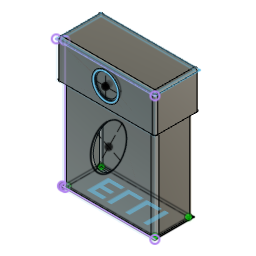
Kartenbox (Autodesk Fusion 360 design; units mm, degrees)
Autodesk Fusion 360 part; units mm, degrees
sketch "Sketch1" plane through (0, 0, 0) normal (0, 0, 1) x (1, 0, 0) in component "Component"
  line L0 (0, 0) -> (69, 0)
  line L1 (69, 0) -> (69, 29)
  line L2 (69, 29) -> (0, 29)
  line L3 (0, 29) -> (0, 0)
  line L4 (2, 27) -> (67, 27)
  line L5 (67, 27) -> (67, 2)
  line L6 (67, 2) -> (2, 2)
  line L7 (2, 2) -> (2, 27)
  line L8 (2, 27) -> (67, 27) construction
  line L9 (67, 27) -> (67, 2) construction
  line L10 (67, 2) -> (2, 2) construction
  line L11 (2, 2) -> (2, 27) construction
  dimension "d46" = 2
  dimension "d47" = 2
  dimension "d48" = 2
  dimension "d49" = 2
  dimension "d80" = 25
  dimension "d81" = 65
  dimension "d98" = 16
  text T0 "ELLI" font "Arial" height 16 bold align centre middle in box 65 x 25 at (2, 27) x (1, 0) y (0, -1) spacing 1 kerned
  constraint horizontal L0
  constraint vertical L1
  constraint horizontal L2
  constraint vertical L3
  constraint coincident L0.start L3.end
  constraint horizontal L4
  constraint vertical L5
  constraint horizontal L6
  constraint vertical L7
  constraint coincident L6.end
  constraint collinear L4 L8
  constraint collinear L5 L9
  measures "d46" distance of L2 L4
  measures "d47" distance of L0 L6
  measures "d48" distance of L3 L7
  measures "d49" distance of L1 L5
  measures "d80" distance of L4 L6
  measures "d81" distance of L5 L7
extrude "Extrude1" add sketch "Sketch1" along normal blind 95 makes body 1 in component "Component"
extrude "Extrude2" add sketch "Sketch1" against normal blind 2 contours L0 L1 L2 L3 | L4 L5 L6 L7 bodies 1 in component "Component"
sketch "Sketch2" plane through (0, 0, 0) normal (0, -1, 0) x (1, 0, 0) in component "Component"
  line L0 (69, -2) -> (69, 95)
  line L1 (69, 95) -> (0, 95)
  line L2 (0, 95) -> (0, -2)
  line L3 (0, -2) -> (69, -2)
  circle A0 centre (34.5, 83) radius 9
  ellipse E0 centre (34.5, 42.5) end of major axis (44.5, 62.6556) minor radius 10
  line L4 (24.5, 22.3444) -> (44.5, 62.6556)
  line L5 (43.4581, 38.0556) -> (25.5419, 46.9444)
  line L6 (2, 0) -> (2, 95)
  line L7 (0, 0) -> (69, 0)
  dimension "d67" = 18
  dimension "d69" = 12
  dimension "d93" = 34.5
  dimension "d94" = 42.5
  dimension "d95" = 45
  dimension "d96" = 20
  dimension "d97" = 10
  constraint coincident E0 L4.start
  constraint coincident E0 L4.end
  constraint coincident E0 L5.start
  constraint coincident E0 L5.end
  constraint vertical A0.centre E0.centre
  measures "d67" diameter of A0
  measures "d69" distance of L1 A0.centre
  measures "d93" distance of L2 A0.centre
  measures "d94" distance of E0.centre L7
  measures "d95" distance of E0
  measures "d97" distance of E0.centre L4.end
extrude "Extrude3" add sketch "Sketch2" along normal blind 1 contours A0 bodies 1 in component "Component"
draft "Draft1" angle 1.5 neutral plane through (0, 0, 95) pull (0, 0, 1) 1 faces at (37.1694, -1, 83.8545) on bodies 1 in component "Component"
extrude "Extrude4" add sketch "Sketch2" along normal blind -29 and the other way blind 30 contours A0 bodies 1 in component "Component"
draft "Draft2" angle 1.5 neutral plane through (0, 0, 95) pull (0, 0, 1) 1 faces at (37.1694, 30, 83.8545) on bodies 1 in component "Component"
extrude "Extrude5" cut sketch "Sketch2" against normal blind 41.885 contours E0 L4 L5 | E0 L4 L5 | E0 L4 L5 | E0 L4 L5 bodies 1 in component "Component"
extrude "Extrude6" cut sketch "Sketch1" against normal blind 5.147 and the other way blind -1.5 text T0 bodies 1 in component "Component"
fillet "Fillet3" radius 3 8 edges at (69, 29, 46.5) (0, 0, 46.5) (0, 29, 46.5) (0, 14.5, -2) (34.5, 29, -2) (34.5, 0, -2) (69, 14.5, -2) (69, 0, 46.5) on bodies 1 in component "Component"
fillet "Fillet1" radius 1.3 20 edges at (26.1091, 29, 79.7455) (26.1091, 0, 86.2545) (34.5, -1.5499, 74) (34.5, 0, 95) (34.5, 29, 95) (69, 14.5, 95) (0, 14.5, 95) (34.5, 30.0786, 92) (2, 27, 47.5) (2, 2, 47.5) (67, 2, 47.5) (67, 27, 47.5) (34.5, 27, 0) (2, 14.5, 0) (34.5, 2, 0) (67, 14.5, 0) (68.1213, 28.1213, 95) (0.8787, 28.1213, 95) (0.8787, 0.8787, 95) (68.1213, 0.8787, 95) on bodies 1 in component "Component"
sketch "Sketch1 (2)" plane through (0, 0, 0) normal (0, 0, 1) x (1, 0, 0) in component "Component'"
  line L0 (1.3, 23.99) -> (70.95, 23.99)
  line L1 (70.95, 23.99) -> (70.95, -5.3725)
  line L2 (70.95, -5.3725) -> (1.3, -5.3725)
  line L3 (1.3, -5.3725) -> (1.3, 23.99)
  line L4 (-0.7, -7.3725) -> (72.95, -7.3725)
  line L5 (72.95, -7.3725) -> (72.95, 25.99)
  line L6 (72.95, 25.99) -> (-0.7, 25.99)
  line L7 (-0.7, 25.99) -> (-0.7, -7.3725)
  dimension "d56" = 2
  dimension "d57" = 2
  dimension "d58" = 2
  dimension "d59" = 2
  dimension "d82" = 29.3625
  dimension "d83" = 69.65
  constraint horizontal L0
  constraint vertical L1
  constraint horizontal L2
  constraint vertical L3
  constraint horizontal L4
  constraint vertical L5
  constraint horizontal L6
  constraint vertical L7
  measures "d56" distance of L1 L5
  measures "d57" distance of L3 L7
  measures "d58" distance of L2 L4
  measures "d59" distance of L0 L6
  measures "d82" distance of L0.end L1.end
  measures "d83" distance of L0.start L0.end
extrude "Extrude1'" add sketch "Sketch1 (2)" against normal blind 27 separate body makes body 2 in component "Component'"
extrude "Extrude2'" add sketch "Sketch1 (2)" along normal blind 2 contours L0 L1 L2 L3 | L4 L5 L6 L7 bodies 2 in component "Component'"
sketch "Sketch2 (2)" plane through (0, -7.3725, 0) normal (0, -1, 0) x (1, 0, 0) in component "Component'"
  line L0 (-0.7, 2) -> (-0.7, -27)
  line L1 (-0.7, -27) -> (72.95, -27)
  line L2 (72.95, -27) -> (72.95, 2)
  line L3 (72.95, 2) -> (-0.7, 2)
  circle A0 centre (36.125, -12.3) radius 9.25
  line L4 (-0.7, 0) -> (72.95, 0)
  ellipse E0 centre (36.125, -12.3) end of major axis (36.125, -2.85) minor radius 9.25
  line L5 (36.125, -21.75) -> (36.125, -2.85)
  line L6 (45.375, -12.3) -> (26.875, -12.3)
  dimension "d64" = 18.5
  dimension "d68" = 12.3
  dimension "d91" = 36.825
  dimension "d104" = 18.9
  constraint concentric A0 E0
  constraint vertical L5
  constraint coincident E0 L5.start
  constraint coincident E0 L5.end
  constraint coincident E0 L6.start
  constraint coincident E0 L6.end
  constraint coincident A0 L6.start
  measures "d64" diameter of A0
  measures "d68" distance of A0.centre L4
  measures "d91" distance of L0 A0.centre
  measures "d104" distance of E0
extrude "Extrude3'" cut sketch "Sketch2 (2)" against normal blind 49.869 contours A0 L5 L6 | A0 E0 L5 | A0 E0 L5 | A0 L5 L6 | A0 L5 L6 | A0 E0 L5 | A0 E0 L5 | A0 L5 L6 bodies 2 in component "Component'"
fillet "Fillet3'" radius 2 8 edges at (72.95, -7.3725, -12.5) (72.95, 9.3088, 2) (36.125, -7.3725, 2) (-0.7, -7.3725, -12.5) (-0.7, 9.3088, 2) (36.125, 25.99, 2) (-0.7, 25.99, -12.5) (72.95, 25.99, -12.5) on bodies 2 in component "Component'"
fillet "Fillet1'" radius 0.99 24 edges at (36.125, -7.3725, -27) (72.95, 9.3088, -27) (36.125, 25.99, -27) (-0.7, 9.3088, -27) (36.125, -5.3725, -27) (1.3, 9.3088, -27) (36.125, 23.99, -27) (70.95, 9.3088, -27) (36.125, -5.3725, 0) (70.95, 9.3088, 0) (36.125, 23.99, 0) (1.3, 9.3088, 0) (36.125, -5.3725, -21.75) (36.125, 23.99, -21.75) (36.125, -7.3725, -21.75) (36.125, 25.99, -21.75) (1.3, -5.3725, -13.5) (1.3, 23.99, -13.5) (70.95, 23.99, -13.5) (70.95, -5.3725, -13.5) (72.3642, 25.4042, -27) (72.3642, -6.7867, -27) (-0.1142, -6.7867, -27) (-0.1142, 25.4042, -27) on bodies 2 in component "Component'"
component "Component" placed x (1, 0, 0) y (0, 1, 0) z (0, 0, 1) at (7.8979, -0.9074, 5.6479)
component "Component'" placed x (1, 0, 0) y (0, 1, 0) z (0, 0, 1) at (6.2574, 4.2307, 100.6479)
equation "d22 = 2.5 mm"
equation "d29 = d22"
equation "d46 = wandstaerke"
equation "d47 = d46"
equation "d48 = d46"
equation "d49 = d48"
equation "d52 = hoehe"
equation "d54 = -wandstaerke"
equation "d56 = wandstaerke"
equation "d57 = d56"
equation "d58 = d57"
equation "d59 = d56"
equation "d60 = -25 mm - wandstaerke"
equation "d62 = wandstaerke"
equation "d72 = -tiefe - ( 2 * wandstaerke )"
equation "d74 = tiefe + 2 * wandstaerke + 1 mm"
equation "d80 = tiefe"
equation "d81 = breite"
equation "d82 = ( tiefe + 2 * wandstaerke ) * 1.0125"
equation "d83 = breite * 1.01 + 2 * wandstaerke"
equation "breite = 65 mm"
equation "tiefe = 25 mm"
equation "hoehe = 95 mm"
equation "wandstaerke = 2 mm"
equation "d91 = ( ( breite * 1.01 ) + ( 4 * wandstaerke ) ) / 2"
equation "d93 = ( breite + 2 * wandstaerke ) / 2"
equation "d94 = hoehe / 2 - 5 mm"
equation "d101 = -wandstaerke + 0.5 mm"
